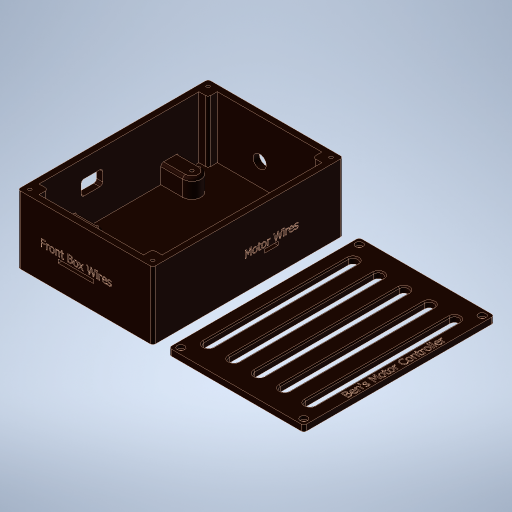
# Autodesk Inventor part: Back Circuit Box
Saved by Autodesk Inventor 2024 (Build 280153000, 153)
## iProperties
Created: 2024-02-09
Part Number: Back Circuit Box
Material: PC/ABS Plastic
Document SubType Name: Modeling
Designer: himmelb
Density: 1.1 g/cm^3
Appearance: Smooth - Dark Brown
Author: himmelb
Autodesk Inventor part; units mm, degrees
(part 1 of 3)
ref_plane "YZ Plane" through (0, 0, 0) normal (1, 0, 0) x (0, 1, 0)
ref_plane "XZ Plane" through (0, 0, 0) normal (0, 1, 0) x (-1, 0, 0)
ref_plane "XY Plane" through (0, 0, 0) normal (0, 0, 1) x (1, 0, 0)
sketch "Sketch1" plane through (0, 0, 0) normal (0, 1, 0) x (-1, 0, 0)
  line L0 (0, 0) -> (110, 0)
  line L1 (110, 0) -> (110, -155)
  line L2 (110, -155) -> (0, -155)
  line L3 (0, -155) -> (0, 0)
  dimension "d0" = 155
  dimension "d1" = 110
  constraints: 8 end point, 2 parallel, 1 horizontal, 1 perpendicular
  measures "d0" distance of L0.end L1.end
  measures "d1" distance of L1.end L2.end
extrude "Extrusion1" add sketch "Sketch1" along normal blind 55
shell "Shell1" thickness 5 removed faces 1 at (-36.6667, 55, -51.6667)
sketch "Sketch2" plane through (0, 0, 0) normal (0, -1, 0) x (1, 0, 0)
  line L0 (12.8693, 0) -> (122.8693, 0)
  line L1 (122.8693, 0) -> (122.8693, -155)
  line L2 (122.8693, -155) -> (12.8693, -155)
  line L3 (12.8693, -155) -> (12.8693, 0)
  point P0 (0, 0)
  dimension "d5" = 110
  dimension "d6" = 155
  constraints: 8 end point, 2 parallel, 1 horizontal, 1 perpendicular
  measures "d5" distance of L1.end L2.end
  measures "d6" distance of L0.end L1.end
extrude "Extrusion2" add sketch "Sketch2" against normal blind 5
sketch "Sketch3" plane through (0, 5, 0) normal (0, 1, 0) x (1, 0, 0)
  line L0 (12.8693, 155) -> (12.8693, 0) projected
  line L1 (105.3693, 18.75) -> (105.3693, 136.25)
  line L2 (112.8693, 136.25) -> (112.8693, 18.75)
  arc A0 (112.8693, 136.25) -> (105.3693, 136.25) centre (109.1193, 136.25) ccw
  arc A1 (105.3693, 18.75) -> (112.8693, 18.75) centre (109.1193, 18.75) ccw
  line L3 (22.8693, 136.25) -> (22.8693, 18.75)
  line L4 (122.8693, 0) -> (122.8693, 155) projected
  circle A2 centre (17.8693, 5) radius 1.335
  circle A3 centre (117.8693, 5) radius 1.335
  circle A4 centre (17.8693, 150) radius 1.335
  circle A5 centre (117.8693, 150) radius 1.335
  line L5 (92.2443, 18.75) -> (92.2443, 136.25)
  arc A6 (92.2443, 136.25) -> (84.7443, 136.25) centre (88.4943, 136.25) ccw
  line L6 (84.7443, 136.25) -> (84.7443, 18.75)
  arc A7 (84.7443, 18.75) -> (92.2443, 18.75) centre (88.4943, 18.75) ccw
  line L7 (71.6193, 18.75) -> (71.6193, 136.25)
  line L8 (122.8693, 155) -> (12.8693, 155) projected
  arc A8 (71.6193, 136.25) -> (67.8693, 140) centre (67.8693, 136.25) ccw
  arc A9 (67.8693, 15) -> (71.6193, 18.75) centre (67.8693, 18.75) ccw
  line L9 (12.8693, 0) -> (122.8693, 0) projected
  line L10 (30.3693, 18.75) -> (30.3693, 136.25)
  line L11 (22.8693, 136.25) -> (22.8693, 18.75)
  arc A10 (30.3693, 136.25) -> (22.8693, 136.25) centre (26.6193, 136.25) ccw
  arc A11 (22.8693, 18.75) -> (30.3693, 18.75) centre (26.6193, 18.75) ccw
  line L12 (43.4943, 18.75) -> (43.4943, 136.25)
  arc A12 (50.9943, 136.25) -> (43.4943, 136.25) centre (47.2443, 136.25) ccw
  line L13 (50.9943, 136.25) -> (50.9943, 18.75)
  arc A13 (43.4943, 18.75) -> (50.9943, 18.75) centre (47.2443, 18.75) ccw
  line L14 (64.1193, 18.75) -> (64.1193, 136.25)
  arc A14 (67.8693, 140) -> (64.1193, 136.25) centre (67.8693, 136.25) ccw
  arc A15 (64.1193, 18.75) -> (67.8693, 15) centre (67.8693, 18.75) ccw
  point P0 (0, 0)
  dimension "d39" = 10
  dimension "d40" = 117.5
  dimension "d41" = 10
  dimension "d45" = 2.67
  dimension "d47" = 5
  dimension "d49" = 5
  dimension "d52" = 5
  dimension "d53" = 5
  dimension "d55" = 2.67
  dimension "d167" = 13.125
  dimension "d168" = 7.5
  dimension "d169" = 13.125
  constraints: 24 point on circle, 22 end point, 16 centre point, 3 vertical
  measures "d39" distance between parallel lines of L4 L2
  measures "d40" distance of L3.start L3.end
  measures "d41" distance between parallel lines of L0 L3
  measures "d45" diameter of A2
  measures "d47" distance from line of A2.centre L0
  measures "d49" distance from line of L4 A3.centre
  measures "d52" distance from line of L0 A4.centre
  measures "d53" distance from line of L4 A5.centre
  measures "d55" diameter of A5
  measures "d167" distance of L1.start L5.start
  measures "d168" diameter of A6
  measures "d169" distance of L6.end L7.start
extrude "Extrusion3" cut sketch "Sketch3" against normal through all contours L1 A0 L2 A1 | A10 L10 A11 L3 | A2 | A3 | A4 | A5 | A7 L6 A6 L5 | A9 A15 L14 A14 A8 L7 | L12 A12 L13 A13
sketch "Sketch4" plane through (0, 5, 0) normal (0, 1, 0) x (1, 0, 0)
  line L0 (115.5683, 32.7918) -> (115.5683, 122.2082) construction
  line L1 (115.5683, 122.2082) -> (120.8693, 122.2082) construction
  line L2 (120.8693, 122.2082) -> (120.8693, 32.7918) construction
  line L3 (120.8693, 32.7918) -> (115.5683, 32.7918) construction
  line L4 (122.8693, 0) -> (122.8693, 155) projected
  spline S0 degree 2 poles (119.4465, 41.7917) (119.8938, 41.7917) (120.5794, 41.4514) (120.8031, 41.1694) knots 0 0 0 1 2 2 2
  spline S1 degree 2 poles (120.8031, 41.1694) (121.0656, 40.829) (121.2893, 40.0559) (121.2893, 39.4433) knots 0 0 0 1 2 2 2
  line L5 (121.2893, 39.4433) -> (121.2893, 37.722)
  line L6 (121.2893, 37.722) -> (115.2893, 37.722)
  line L7 (115.2893, 37.722) -> (115.2893, 39.312)
  spline S2 degree 2 poles (115.2893, 39.312) (115.2893, 39.9538) (115.3719, 40.5956) (115.5324, 40.8874) knots 0 0 0 1 2 2 2
  spline S3 degree 2 poles (115.5324, 40.8874) (115.7026, 41.2131) (116.2617, 41.5097) (116.641, 41.5097) knots 0 0 0 1 2 2 2
  spline S4 degree 2 poles (116.641, 41.5097) (117.064, 41.5097) (117.735, 41.0624) (117.9246, 40.6686) knots 0 0 0 1 2 2 2
  line L8 (117.9246, 40.6686) -> (117.9538, 40.6686)
  spline S5 degree 2 poles (117.9538, 40.6686) (118.0997, 41.2034) (118.8728, 41.7917) (119.4465, 41.7917) knots 0 0 0 1 2 2 2
  spline S6 degree 2 poles (119.4805, 40.9603) (119.1402, 40.9603) (118.7026, 40.7658) (118.547, 40.4741) knots 0 0 0 1 2 2 2
  spline S7 degree 2 poles (118.547, 40.4741) (118.4497, 40.2844) (118.3914, 39.8371) (118.3914, 39.4238) knots 0 0 0 1 2 2 2
  line L9 (118.3914, 39.4238) -> (118.3914, 38.5194)
  line L10 (118.3914, 38.5194) -> (120.6086, 38.5194)
  line L11 (120.6086, 38.5194) -> (120.6086, 39.1661)
  spline S8 degree 2 poles (120.6086, 39.1661) (120.6086, 39.6912) (120.5113, 40.2942) (120.3557, 40.5275) knots 0 0 0 1 2 2 2
  spline S9 degree 2 poles (120.3557, 40.5275) (120.1953, 40.7512) (119.7966, 40.9603) (119.4805, 40.9603) knots 0 0 0 1 2 2 2
  spline S10 degree 2 poles (116.7528, 40.6783) (116.5389, 40.6783) (116.218, 40.5324) (116.1256, 40.372) knots 0 0 0 1 2 2 2
  spline S11 degree 2 poles (116.1256, 40.372) (116.0186, 40.1775) (115.97, 39.7058) (115.97, 39.2828) knots 0 0 0 1 2 2 2
  line L12 (115.97, 39.2828) -> (115.97, 38.5194)
  line L13 (115.97, 38.5194) -> (117.7253, 38.5194)
  line L14 (117.7253, 38.5194) -> (117.7253, 39.4238)
  spline S12 degree 2 poles (117.7253, 39.4238) (117.7253, 39.7982) (117.6475, 40.1532) (117.5259, 40.3428) knots 0 0 0 1 2 2 2
  spline S13 degree 2 poles (117.5259, 40.3428) (117.4092, 40.5275) (117.0348, 40.6783) (116.7528, 40.6783) knots 0 0 0 1 2 2 2
  spline S14 degree 2 poles (121.3914, 44.4805) (121.3914, 43.4011) (120.1807, 42.2147) (119.0624, 42.2147) knots 0 0 0 1 2 2 2
  spline S15 degree 2 poles (119.0624, 42.2147) (117.9635, 42.2147) (116.6604, 43.3671) (116.6604, 44.2958) knots 0 0 0 1 2 2 2
  spline S16 degree 2 poles (116.6604, 44.2958) (116.6604, 44.7139) (116.9036, 45.3606) (117.1612, 45.5989) knots 0 0 0 1 2 2 2
  spline S17 degree 2 poles (117.1612, 45.5989) (117.4189, 45.842) (118.1629, 46.0997) (118.7026, 46.0997) knots 0 0 0 1 2 2 2
  line L15 (118.7026, 46.0997) -> (119.1159, 46.0997)
  line L16 (119.1159, 46.0997) -> (119.1159, 42.983)
  spline S18 degree 2 poles (119.1159, 42.983) (119.8987, 42.983) (120.7301, 43.7707) (120.7301, 44.4708) knots 0 0 0 1 2 2 2
  spline S19 degree 2 poles (120.7301, 44.4708) (120.7301, 44.7188) (120.6183, 45.2002) (120.5308, 45.3946) knots 0 0 0 1 2 2 2
  spline S20 degree 2 poles (120.5308, 45.3946) (120.4335, 45.5989) (120.2634, 45.8809) (120.1856, 45.9733) knots 0 0 0 1 2 2 2
  line L17 (120.1856, 45.9733) -> (120.1856, 46.017)
  line L18 (120.1856, 46.017) -> (121.0121, 46.017)
  spline S21 degree 2 poles (121.0121, 46.017) (121.0656, 45.8857) (121.2212, 45.487) (121.265, 45.3314) knots 0 0 0 1 2 2 2
  spline S22 degree 2 poles (121.265, 45.3314) (121.3282, 45.1126) (121.3914, 44.7528) (121.3914, 44.4805) knots 0 0 0 1 2 2 2
  spline S23 degree 2 poles (118.5373, 45.3606) (118.2309, 45.3509) (117.7836, 45.2245) (117.6329, 45.1029) knots 0 0 0 1 2 2 2
  spline S24 degree 2 poles (117.6329, 45.1029) (117.4627, 44.9716) (117.2828, 44.5583) (117.2828, 44.252) knots 0 0 0 1 2 2 2
  spline S25 degree 2 poles (117.2828, 44.252) (117.2828, 43.9506) (117.4627, 43.5275) (117.6377, 43.3525) knots 0 0 0 1 2 2 2
  spline S26 degree 2 poles (117.6377, 43.3525) (117.8177, 43.1823) (118.2504, 43.0073) (118.5373, 42.983) knots 0 0 0 1 2 2 2
  line L19 (118.5373, 42.983) -> (118.5373, 45.3606)
  line L20 (121.2893, 50.4028) -> (121.2893, 49.6442)
  line L21 (121.2893, 49.6442) -> (118.722, 49.6442)
  spline S27 degree 2 poles (118.722, 49.6442) (118.4108, 49.6442) (117.876, 49.5859) (117.7155, 49.4984) knots 0 0 0 1 2 2 2
  spline S28 degree 2 poles (117.7155, 49.4984) (117.5454, 49.406) (117.38, 49.0754) (117.38, 48.7934) knots 0 0 0 1 2 2 2
  spline S29 degree 2 poles (117.38, 48.7934) (117.38, 48.5113) (117.6815, 47.9133) (117.9246, 47.6264) knots 0 0 0 1 2 2 2
  line L22 (117.9246, 47.6264) -> (121.2893, 47.6264)
  line L23 (121.2893, 47.6264) -> (121.2893, 46.8679)
  line L24 (121.2893, 46.8679) -> (116.7869, 46.8679)
  line L25 (116.7869, 46.8679) -> (116.7869, 47.6264)
  line L26 (116.7869, 47.6264) -> (117.2877, 47.6264)
  spline S30 degree 2 poles (117.2877, 47.6264) (116.9813, 47.9668) (116.6604, 48.6232) (116.6604, 48.9927) knots 0 0 0 1 2 2 2
  spline S31 degree 2 poles (116.6604, 48.9927) (116.6604, 49.654) (117.5356, 50.4028) (118.3671, 50.4028) knots 0 0 0 1 2 2 2
  line L27 (118.3671, 50.4028) -> (121.2893, 50.4028)
  line L28 (115.0219, 52.2358) -> (117.3557, 52.0608)
  line L29 (117.3557, 52.0608) -> (117.3557, 51.5162)
  line L30 (117.3557, 51.5162) -> (115.0219, 51.3412)
  line L31 (115.0219, 51.3412) -> (115.0219, 52.2358)
  spline S32 degree 2 poles (121.3963, 54.4238) (121.3963, 53.9716) (121.1531, 53.1888) (121.017, 52.9311) knots 0 0 0 1 2 2 2
  line L32 (121.017, 52.9311) -> (120.1661, 52.9311)
  line L33 (120.1661, 52.9311) -> (120.1661, 52.97)
  spline S33 degree 2 poles (120.1661, 52.97) (120.2439, 53.0673) (120.4287, 53.3298) (120.5308, 53.5486) knots 0 0 0 1 2 2 2
  spline S34 degree 2 poles (120.5308, 53.5486) (120.6232, 53.7382) (120.7593, 54.205) (120.7593, 54.453) knots 0 0 0 1 2 2 2
  spline S35 degree 2 poles (120.7593, 54.453) (120.7593, 54.6329) (120.6766, 55.0462) (120.6086, 55.1434) knots 0 0 0 1 2 2 2
  spline S36 degree 2 poles (120.6086, 55.1434) (120.5162, 55.2844) (120.3071, 55.4109) (120.0932, 55.4109) knots 0 0 0 1 2 2 2
  spline S37 degree 2 poles (120.0932, 55.4109) (119.8258, 55.4109) (119.5486, 55.1191) (119.4562, 54.7447) knots 0 0 0 1 2 2 2
  spline S38 degree 2 poles (119.4562, 54.7447) (119.4222, 54.5989) (119.3249, 54.1321) (119.2715, 53.9327) knots 0 0 0 1 2 2 2
  spline S39 degree 2 poles (119.2715, 53.9327) (119.1207, 53.4173) (118.4984, 52.9506) (118.0559, 52.9506) knots 0 0 0 1 2 2 2
  spline S40 degree 2 poles (118.0559, 52.9506) (117.4433, 52.9506) (116.6799, 53.8695) (116.6799, 54.628) knots 0 0 0 1 2 2 2
  spline S41 degree 2 poles (116.6799, 54.628) (116.6799, 55.0024) (116.8647, 55.7609) (117.0057, 56.0186) knots 0 0 0 1 2 2 2
  line L34 (117.0057, 56.0186) -> (117.8177, 56.0186)
  line L35 (117.8177, 56.0186) -> (117.8177, 55.9797)
  spline S42 degree 2 poles (117.8177, 55.9797) (117.5843, 55.688) (117.3168, 54.9781) (117.3168, 54.6134) knots 0 0 0 1 2 2 2
  spline S43 degree 2 poles (117.3168, 54.6134) (117.3168, 54.2391) (117.6329, 53.7237) (117.9489, 53.7237) knots 0 0 0 1 2 2 2
  spline S44 degree 2 poles (117.9489, 53.7237) (118.2358, 53.7237) (118.513, 54.03) (118.6005, 54.3703) knots 0 0 0 1 2 2 2
  spline S45 degree 2 poles (118.6005, 54.3703) (118.6442, 54.5357) (118.7318, 54.9538) (118.7852, 55.1823) knots 0 0 0 1 2 2 2
  spline S46 degree 2 poles (118.7852, 55.1823) (118.9117, 55.6783) (119.4903, 56.184) (119.9911, 56.184) knots 0 0 0 1 2 2 2
  spline S47 degree 2 poles (119.9911, 56.184) (120.2828, 56.184) (120.7982, 55.9554) (120.9878, 55.7318) knots 0 0 0 1 2 2 2
  spline S48 degree 2 poles (120.9878, 55.7318) (121.1872, 55.4935) (121.3963, 54.8857) (121.3963, 54.4238) knots 0 0 0 1 2 2 2
  line L36 (121.2893, 64.6686) -> (121.2893, 63.8711)
  line L37 (121.2893, 63.8711) -> (116.1207, 63.8711)
  line L38 (116.1207, 63.8711) -> (119.6361, 62.3055)
  line L39 (119.6361, 62.3055) -> (119.6361, 61.8193)
  line L40 (119.6361, 61.8193) -> (116.1207, 60.2682)
  line L41 (116.1207, 60.2682) -> (121.2893, 60.2682)
  line L42 (121.2893, 60.2682) -> (121.2893, 59.5243)
  line L43 (121.2893, 59.5243) -> (115.2893, 59.5243)
  line L44 (115.2893, 59.5243) -> (115.2893, 60.6134)
  line L45 (115.2893, 60.6134) -> (118.6296, 62.111)
  line L46 (118.6296, 62.111) -> (115.2893, 63.56)
  line L47 (115.2893, 63.56) -> (115.2893, 64.6686)
  line L48 (115.2893, 64.6686) -> (121.2893, 64.6686)
  spline S49 degree 2 poles (119.0381, 69.5259) (120.1758, 69.5259) (121.4157, 68.4319) (121.4157, 67.5178) knots 0 0 0 1 2 2 2
  spline S50 degree 2 poles (121.4157, 67.5178) (121.4157, 66.5794) (120.1369, 65.5049) (119.0381, 65.5049) knots 0 0 0 1 2 2 2
  spline S51 degree 2 poles (119.0381, 65.5049) (117.91, 65.5049) (116.6604, 66.6134) (116.6604, 67.5178) knots 0 0 0 1 2 2 2
  spline S52 degree 2 poles (116.6604, 67.5178) (116.6604, 68.4319) (117.9052, 69.5259) (119.0381, 69.5259) knots 0 0 0 1 2 2 2
  spline S53 degree 2 poles (119.0381, 68.7431) (118.1629, 68.7431) (117.312, 68.1062) (117.312, 67.5178) knots 0 0 0 1 2 2 2
  spline S54 degree 2 poles (117.312, 67.5178) (117.312, 66.9295) (118.1629, 66.2877) (119.0381, 66.2877) knots 0 0 0 1 2 2 2
  spline S55 degree 2 poles (119.0381, 66.2877) (119.889, 66.2877) (120.7642, 66.9295) (120.7642, 67.5178) knots 0 0 0 1 2 2 2
  spline S56 degree 2 poles (120.7642, 67.5178) (120.7642, 68.1013) (119.9036, 68.7431) (119.0381, 68.7431) knots 0 0 0 1 2 2 2
  spline S57 degree 2 poles (121.3768, 71.6653) (121.3768, 71.0478) (120.6718, 70.3525) (119.9084, 70.3525) knots 0 0 0 1 2 2 2
  line L49 (119.9084, 70.3525) -> (117.4141, 70.3525)
  line L50 (117.4141, 70.3525) -> (117.4141, 69.842)
  line L51 (117.4141, 69.842) -> (116.7869, 69.842)
  line L52 (116.7869, 69.842) -> (116.7869, 70.3525)
  line L53 (116.7869, 70.3525) -> (115.4935, 70.3525)
  line L54 (115.4935, 70.3525) -> (115.4935, 71.111)
  line L55 (115.4935, 71.111) -> (116.7869, 71.111)
  line L56 (116.7869, 71.111) -> (116.7869, 72.5065)
  line L57 (116.7869, 72.5065) -> (117.4141, 72.5065)
  line L58 (117.4141, 72.5065) -> (117.4141, 71.111)
  line L59 (117.4141, 71.111) -> (119.5583, 71.111)
  spline S58 degree 2 poles (119.5583, 71.111) (119.8987, 71.111) (120.2731, 71.1353) (120.4335, 71.218) knots 0 0 0 1 2 2 2
  spline S59 degree 2 poles (120.4335, 71.218) (120.5745, 71.2861) (120.7155, 71.5924) (120.7155, 71.8549) knots 0 0 0 1 2 2 2
  spline S60 degree 2 poles (120.7155, 71.8549) (120.7155, 72.0397) (120.6037, 72.3849) (120.5697, 72.4627) knots 0 0 0 1 2 2 2
  line L60 (120.5697, 72.4627) -> (120.5697, 72.5065)
  line L61 (120.5697, 72.5065) -> (121.2504, 72.5065)
  spline S61 degree 2 poles (121.2504, 72.5065) (121.3087, 72.2925) (121.3768, 71.8549) (121.3768, 71.6653) knots 0 0 0 1 2 2 2
  spline S62 degree 2 poles (119.0381, 76.7658) (120.1758, 76.7658) (121.4157, 75.6718) (121.4157, 74.7577) knots 0 0 0 1 2 2 2
  spline S63 degree 2 poles (121.4157, 74.7577) (121.4157, 73.8193) (120.1369, 72.7447) (119.0381, 72.7447) knots 0 0 0 1 2 2 2
  spline S64 degree 2 poles (119.0381, 72.7447) (117.91, 72.7447) (116.6604, 73.8533) (116.6604, 74.7577) knots 0 0 0 1 2 2 2
  spline S65 degree 2 poles (116.6604, 74.7577) (116.6604, 75.6718) (117.9052, 76.7658) (119.0381, 76.7658) knots 0 0 0 1 2 2 2
  spline S66 degree 2 poles (119.0381, 75.983) (118.1629, 75.983) (117.312, 75.346) (117.312, 74.7577) knots 0 0 0 1 2 2 2
  spline S67 degree 2 poles (117.312, 74.7577) (117.312, 74.1694) (118.1629, 73.5275) (119.0381, 73.5275) knots 0 0 0 1 2 2 2
  spline S68 degree 2 poles (119.0381, 73.5275) (119.889, 73.5275) (120.7642, 74.1694) (120.7642, 74.7577) knots 0 0 0 1 2 2 2
  spline S69 degree 2 poles (120.7642, 74.7577) (120.7642, 75.3412) (119.9036, 75.983) (119.0381, 75.983) knots 0 0 0 1 2 2 2
  line L62 (117.5988, 79.9311) -> (117.5988, 79.8922)
  spline S70 degree 2 poles (117.5988, 79.8922) (117.5745, 79.8047) (117.5648, 79.6151) (117.5648, 79.4838) knots 0 0 0 1 2 2 2
  spline S71 degree 2 poles (117.5648, 79.4838) (117.5648, 79.1775) (117.8322, 78.5746) (118.0948, 78.3023) knots 0 0 0 1 2 2 2
  line L63 (118.0948, 78.3023) -> (121.2893, 78.3023)
  line L64 (121.2893, 78.3023) -> (121.2893, 77.5438)
  line L65 (121.2893, 77.5438) -> (116.7869, 77.5438)
  line L66 (116.7869, 77.5438) -> (116.7869, 78.3023)
  line L67 (116.7869, 78.3023) -> (117.4578, 78.3023)
  spline S72 degree 2 poles (117.4578, 78.3023) (117.0883, 78.7156) (116.7869, 79.3331) (116.7869, 79.6248) knots 0 0 0 1 2 2 2
  spline S73 degree 2 poles (116.7869, 79.6248) (116.7869, 79.7415) (116.7966, 79.8582) (116.8112, 79.9311) knots 0 0 0 1 2 2 2
  line L68 (116.8112, 79.9311) -> (117.5988, 79.9311)
  spline S74 degree 2 poles (121.3963, 85.4984) (121.3963, 84.9149) (121.0024, 83.9279) (120.6086, 83.5681) knots 0 0 0 1 2 2 2
  spline S75 degree 2 poles (120.6086, 83.5681) (120.2196, 83.2083) (119.0527, 82.8144) (118.2941, 82.8144) knots 0 0 0 1 2 2 2
  spline S76 degree 2 poles (118.2941, 82.8144) (117.5405, 82.8144) (116.4222, 83.1985) (116.0089, 83.5632) knots 0 0 0 1 2 2 2
  spline S77 degree 2 poles (116.0089, 83.5632) (115.6053, 83.923) (115.1823, 84.9052) (115.1823, 85.513) knots 0 0 0 1 2 2 2
  spline S78 degree 2 poles (115.1823, 85.513) (115.1823, 85.8144) (115.2698, 86.3444) (115.3379, 86.5681) knots 0 0 0 1 2 2 2
  spline S79 degree 2 poles (115.3379, 86.5681) (115.4011, 86.7626) (115.581, 87.1661) (115.688, 87.3655) knots 0 0 0 1 2 2 2
  line L69 (115.688, 87.3655) -> (116.6507, 87.3655)
  line L70 (116.6507, 87.3655) -> (116.6507, 87.3023)
  spline S80 degree 2 poles (116.6507, 87.3023) (116.5535, 87.1953) (116.2812, 86.8647) (116.1499, 86.6264) knots 0 0 0 1 2 2 2
  spline S81 degree 2 poles (116.1499, 86.6264) (116.0235, 86.3979) (115.863, 85.8582) (115.863, 85.5081) knots 0 0 0 1 2 2 2
  spline S82 degree 2 poles (115.863, 85.5081) (115.863, 85.124) (116.1791, 84.4384) (116.4805, 84.1807) knots 0 0 0 1 2 2 2
  spline S83 degree 2 poles (116.4805, 84.1807) (116.7869, 83.9279) (117.7155, 83.6459) (118.2941, 83.6459) knots 0 0 0 1 2 2 2
  spline S84 degree 2 poles (118.2941, 83.6459) (118.9117, 83.6459) (119.8014, 83.9425) (120.1078, 84.2002) knots 0 0 0 1 2 2 2
  spline S85 degree 2 poles (120.1078, 84.2002) (120.4044, 84.453) (120.7058, 85.1288) (120.7058, 85.5081) knots 0 0 0 1 2 2 2
  spline S86 degree 2 poles (120.7058, 85.5081) (120.7058, 85.8533) (120.5356, 86.4417) (120.4092, 86.6702) knots 0 0 0 1 2 2 2
  spline S87 degree 2 poles (120.4092, 86.6702) (120.2828, 86.889) (120.0202, 87.2147) (119.9279, 87.3071) knots 0 0 0 1 2 2 2
  line L71 (119.9279, 87.3071) -> (119.9279, 87.3655)
  line L72 (119.9279, 87.3655) -> (120.8809, 87.3655)
  spline S88 degree 2 poles (120.8809, 87.3655) (120.9732, 87.1661) (121.1434, 86.816) (121.2212, 86.5681) knots 0 0 0 1 2 2 2
  spline S89 degree 2 poles (121.2212, 86.5681) (121.3087, 86.3055) (121.3963, 85.8582) (121.3963, 85.4984) knots 0 0 0 1 2 2 2
  spline S90 degree 2 poles (119.0381, 91.7512) (120.1758, 91.7512) (121.4157, 90.6572) (121.4157, 89.7431) knots 0 0 0 1 2 2 2
  spline S91 degree 2 poles (121.4157, 89.7431) (121.4157, 88.8047) (120.1369, 87.7301) (119.0381, 87.7301) knots 0 0 0 1 2 2 2
  spline S92 degree 2 poles (119.0381, 87.7301) (117.91, 87.7301) (116.6604, 88.8387) (116.6604, 89.7431) knots 0 0 0 1 2 2 2
  spline S93 degree 2 poles (116.6604, 89.7431) (116.6604, 90.6572) (117.9052, 91.7512) (119.0381, 91.7512) knots 0 0 0 1 2 2 2
  spline S94 degree 2 poles (119.0381, 90.9684) (118.1629, 90.9684) (117.312, 90.3314) (117.312, 89.7431) knots 0 0 0 1 2 2 2
  spline S95 degree 2 poles (117.312, 89.7431) (117.312, 89.1548) (118.1629, 88.513) (119.0381, 88.513) knots 0 0 0 1 2 2 2
  spline S96 degree 2 poles (119.0381, 88.513) (119.889, 88.513) (120.7642, 89.1548) (120.7642, 89.7431) knots 0 0 0 1 2 2 2
  spline S97 degree 2 poles (120.7642, 89.7431) (120.7642, 90.3266) (119.9036, 90.9684) (119.0381, 90.9684) knots 0 0 0 1 2 2 2
  line L73 (121.2893, 96.064) -> (121.2893, 95.3055)
  line L74 (121.2893, 95.3055) -> (118.722, 95.3055)
  spline S98 degree 2 poles (118.722, 95.3055) (118.4108, 95.3055) (117.876, 95.2472) (117.7155, 95.1596) knots 0 0 0 1 2 2 2
  spline S99 degree 2 poles (117.7155, 95.1596) (117.5454, 95.0673) (117.38, 94.7366) (117.38, 94.4546) knots 0 0 0 1 2 2 2
  spline S100 degree 2 poles (117.38, 94.4546) (117.38, 94.1726) (117.6815, 93.5746) (117.9246, 93.2877) knots 0 0 0 1 2 2 2
  line L75 (117.9246, 93.2877) -> (121.2893, 93.2877)
  line L76 (121.2893, 93.2877) -> (121.2893, 92.5292)
  line L77 (121.2893, 92.5292) -> (116.7869, 92.5292)
  line L78 (116.7869, 92.5292) -> (116.7869, 93.2877)
  line L79 (116.7869, 93.2877) -> (117.2877, 93.2877)
  spline S101 degree 2 poles (117.2877, 93.2877) (116.9813, 93.628) (116.6604, 94.2844) (116.6604, 94.654) knots 0 0 0 1 2 2 2
  spline S102 degree 2 poles (116.6604, 94.654) (116.6604, 95.3152) (117.5356, 96.064) (118.3671, 96.064) knots 0 0 0 1 2 2 2
  line L80 (118.3671, 96.064) -> (121.2893, 96.064)
  spline S103 degree 2 poles (121.3768, 98.4903) (121.3768, 97.8728) (120.6718, 97.1775) (119.9084, 97.1775) knots 0 0 0 1 2 2 2
  line L81 (119.9084, 97.1775) -> (117.4141, 97.1775)
  line L82 (117.4141, 97.1775) -> (117.4141, 96.6669)
  line L83 (117.4141, 96.6669) -> (116.7869, 96.6669)
  line L84 (116.7869, 96.6669) -> (116.7869, 97.1775)
  line L85 (116.7869, 97.1775) -> (115.4935, 97.1775)
  line L86 (115.4935, 97.1775) -> (115.4935, 97.936)
  line L87 (115.4935, 97.936) -> (116.7869, 97.936)
  line L88 (116.7869, 97.936) -> (116.7869, 99.3314)
  line L89 (116.7869, 99.3314) -> (117.4141, 99.3314)
  line L90 (117.4141, 99.3314) -> (117.4141, 97.936)
  line L91 (117.4141, 97.936) -> (119.5583, 97.936)
  spline S104 degree 2 poles (119.5583, 97.936) (119.8987, 97.936) (120.2731, 97.9603) (120.4335, 98.0429) knots 0 0 0 1 2 2 2
  spline S105 degree 2 poles (120.4335, 98.0429) (120.5745, 98.111) (120.7155, 98.4173) (120.7155, 98.6799) knots 0 0 0 1 2 2 2
  spline S106 degree 2 poles (120.7155, 98.6799) (120.7155, 98.8647) (120.6037, 99.2099) (120.5697, 99.2877) knots 0 0 0 1 2 2 2
  line L92 (120.5697, 99.2877) -> (120.5697, 99.3314)
  line L93 (120.5697, 99.3314) -> (121.2504, 99.3314)
  spline S107 degree 2 poles (121.2504, 99.3314) (121.3087, 99.1175) (121.3768, 98.6799) (121.3768, 98.4903) knots 0 0 0 1 2 2 2
  line L94 (117.5988, 102.278) -> (117.5988, 102.2391)
  spline S108 degree 2 poles (117.5988, 102.2391) (117.5745, 102.1515) (117.5648, 101.9619) (117.5648, 101.8306) knots 0 0 0 1 2 2 2
  spline S109 degree 2 poles (117.5648, 101.8306) (117.5648, 101.5243) (117.8322, 100.9214) (118.0948, 100.6491) knots 0 0 0 1 2 2 2
  line L95 (118.0948, 100.6491) -> (121.2893, 100.6491)
  line L96 (121.2893, 100.6491) -> (121.2893, 99.8906)
  line L97 (121.2893, 99.8906) -> (116.7869, 99.8906)
  line L98 (116.7869, 99.8906) -> (116.7869, 100.6491)
  line L99 (116.7869, 100.6491) -> (117.4578, 100.6491)
  spline S110 degree 2 poles (117.4578, 100.6491) (117.0883, 101.0624) (116.7869, 101.6799) (116.7869, 101.9716) knots 0 0 0 1 2 2 2
  spline S111 degree 2 poles (116.7869, 101.9716) (116.7869, 102.0883) (116.7966, 102.205) (116.8112, 102.278) knots 0 0 0 1 2 2 2
  line L100 (116.8112, 102.278) -> (117.5988, 102.278)
  spline S112 degree 2 poles (119.0381, 106.5664) (120.1758, 106.5664) (121.4157, 105.4724) (121.4157, 104.5583) knots 0 0 0 1 2 2 2
  spline S113 degree 2 poles (121.4157, 104.5583) (121.4157, 103.6199) (120.1369, 102.5454) (119.0381, 102.5454) knots 0 0 0 1 2 2 2
  spline S114 degree 2 poles (119.0381, 102.5454) (117.91, 102.5454) (116.6604, 103.654) (116.6604, 104.5583) knots 0 0 0 1 2 2 2
  spline S115 degree 2 poles (116.6604, 104.5583) (116.6604, 105.4724) (117.9052, 106.5664) (119.0381, 106.5664) knots 0 0 0 1 2 2 2
  spline S116 degree 2 poles (119.0381, 105.7836) (118.1629, 105.7836) (117.312, 105.1467) (117.312, 104.5583) knots 0 0 0 1 2 2 2
  spline S117 degree 2 poles (117.312, 104.5583) (117.312, 103.97) (118.1629, 103.3282) (119.0381, 103.3282) knots 0 0 0 1 2 2 2
  spline S118 degree 2 poles (119.0381, 103.3282) (119.889, 103.3282) (120.7642, 103.97) (120.7642, 104.5583) knots 0 0 0 1 2 2 2
  spline S119 degree 2 poles (120.7642, 104.5583) (120.7642, 105.1418) (119.9036, 105.7836) (119.0381, 105.7836) knots 0 0 0 1 2 2 2
  line L101 (121.2893, 108.1175) -> (121.2893, 107.359)
  line L102 (121.2893, 107.359) -> (115.0219, 107.359)
  line L103 (115.0219, 107.359) -> (115.0219, 108.1175)
  line L104 (115.0219, 108.1175) -> (121.2893, 108.1175)
  line L105 (121.2893, 110.0041) -> (121.2893, 109.2455)
  line L106 (121.2893, 109.2455) -> (115.0219, 109.2455)
  line L107 (115.0219, 109.2455) -> (115.0219, 110.0041)
  line L108 (115.0219, 110.0041) -> (121.2893, 110.0041)
  spline S120 degree 2 poles (121.3914, 113.0721) (121.3914, 111.9927) (120.1807, 110.8063) (119.0624, 110.8063) knots 0 0 0 1 2 2 2
  spline S121 degree 2 poles (119.0624, 110.8063) (117.9635, 110.8063) (116.6604, 111.9587) (116.6604, 112.8874) knots 0 0 0 1 2 2 2
  spline S122 degree 2 poles (116.6604, 112.8874) (116.6604, 113.3055) (116.9036, 113.9522) (117.1612, 114.1904) knots 0 0 0 1 2 2 2
  spline S123 degree 2 poles (117.1612, 114.1904) (117.4189, 114.4335) (118.1629, 114.6912) (118.7026, 114.6912) knots 0 0 0 1 2 2 2
  line L109 (118.7026, 114.6912) -> (119.1159, 114.6912)
  line L110 (119.1159, 114.6912) -> (119.1159, 111.5746)
  spline S124 degree 2 poles (119.1159, 111.5746) (119.8987, 111.5746) (120.7301, 112.3622) (120.7301, 113.0624) knots 0 0 0 1 2 2 2
  spline S125 degree 2 poles (120.7301, 113.0624) (120.7301, 113.3104) (120.6183, 113.7917) (120.5308, 113.9862) knots 0 0 0 1 2 2 2
  spline S126 degree 2 poles (120.5308, 113.9862) (120.4335, 114.1904) (120.2634, 114.4724) (120.1856, 114.5648) knots 0 0 0 1 2 2 2
  line L111 (120.1856, 114.5648) -> (120.1856, 114.6086)
  line L112 (120.1856, 114.6086) -> (121.0121, 114.6086)
  spline S127 degree 2 poles (121.0121, 114.6086) (121.0656, 114.4773) (121.2212, 114.0786) (121.265, 113.923) knots 0 0 0 1 2 2 2
  spline S128 degree 2 poles (121.265, 113.923) (121.3282, 113.7042) (121.3914, 113.3444) (121.3914, 113.0721) knots 0 0 0 1 2 2 2
  spline S129 degree 2 poles (118.5373, 113.9522) (118.2309, 113.9425) (117.7836, 113.816) (117.6329, 113.6945) knots 0 0 0 1 2 2 2
  spline S130 degree 2 poles (117.6329, 113.6945) (117.4627, 113.5632) (117.2828, 113.1499) (117.2828, 112.8436) knots 0 0 0 1 2 2 2
  spline S131 degree 2 poles (117.2828, 112.8436) (117.2828, 112.5421) (117.4627, 112.1191) (117.6377, 111.9441) knots 0 0 0 1 2 2 2
  spline S132 degree 2 poles (117.6377, 111.9441) (117.8177, 111.7739) (118.2504, 111.5989) (118.5373, 111.5746) knots 0 0 0 1 2 2 2
  line L113 (118.5373, 111.5746) -> (118.5373, 113.9522)
  line L114 (117.5988, 117.8468) -> (117.5988, 117.8079)
  spline S133 degree 2 poles (117.5988, 117.8079) (117.5745, 117.7204) (117.5648, 117.5308) (117.5648, 117.3995) knots 0 0 0 1 2 2 2
  spline S134 degree 2 poles (117.5648, 117.3995) (117.5648, 117.0932) (117.8322, 116.4903) (118.0948, 116.218) knots 0 0 0 1 2 2 2
  line L115 (118.0948, 116.218) -> (121.2893, 116.218)
  line L116 (121.2893, 116.218) -> (121.2893, 115.4595)
  line L117 (121.2893, 115.4595) -> (116.7869, 115.4595)
  line L118 (116.7869, 115.4595) -> (116.7869, 116.218)
  line L119 (116.7869, 116.218) -> (117.4578, 116.218)
  spline S135 degree 2 poles (117.4578, 116.218) (117.0883, 116.6313) (116.7869, 117.2488) (116.7869, 117.5405) knots 0 0 0 1 2 2 2
  spline S136 degree 2 poles (116.7869, 117.5405) (116.7869, 117.6572) (116.7966, 117.7739) (116.8112, 117.8468) knots 0 0 0 1 2 2 2
  line L120 (116.8112, 117.8468) -> (117.5988, 117.8468)
  point P0 (0, 0)
  point P1 (120.8693, 77.5)
  point P2 (122.8693, 77.5)
  point P3 (120.8693, 77.5)
  point P4 (122.8693, 77.5)
  dimension "d59" = 2
  dimension "d61" = 0
  constraints: 3 midpoint, 1 coincident, 2 other
  measures "d59" distance between parallel lines of L4 L2
  measures "d61" vertical distance of point (122.869, 77.5) point (120.869, 77.5)
extrude "Extrusion4" cut sketch "Sketch4" against normal blind 1.5
sketch "Sketch5" plane through (0, 5, 0) normal (0, 1, 0) x (1, 0, 0)
  circle A0 centre (17.8693, 5) radius 1.335 projected
  circle A1 centre (17.8693, 5) radius 3
  circle A2 centre (17.8693, 150) radius 1.335 projected
  circle A3 centre (17.8693, 150) radius 3
  circle A4 centre (117.8693, 150) radius 1.335 projected
  circle A5 centre (117.8693, 150) radius 3
  circle A6 centre (117.8693, 5) radius 1.335 projected
  circle A7 centre (117.8693, 5) radius 3
  point P0 (0, 0)
  dimension "d66" = 6
  dimension "d67" = 6
  dimension "d68" = 6
  dimension "d69" = 6
  constraints: 4 centre point, 4 coincident
  measures "d66" diameter of A1
  measures "d67" diameter of A7
  measures "d68" diameter of A5
  measures "d69" diameter of A3
extrude "Extrusion5" cut sketch "Sketch5" against normal blind 2.7 contours A0 | A1 | A2 | A3 | A4 | A5 | A6 | A7
sketch "Sketch6" plane through (-105, 5, -150) normal (0, 1, 0) x (1, 0, 0)
  line L0 (0, 0) -> (100, 0) projected
  line L1 (0, 0) -> (7.5, 0)
  line L2 (7.5, 0) -> (7.5, -7.5)
  line L3 (7.5, -7.5) -> (0, -7.5)
  line L4 (0, -7.5) -> (0, 0)
  line L5 (0, -145) -> (0, 0) projected
  line L6 (100, 0) -> (0, 0)
  line L7 (100, 0) -> (92.5, 0)
  line L8 (92.5, 0) -> (92.5, -7.5)
  line L9 (92.5, -7.5) -> (100, -7.5)
  line L10 (100, -145) -> (100, 0)
  line L11 (100, 0) -> (100, -7.5)
  line L12 (0, -145) -> (7.5, -145)
  line L13 (7.5, -145) -> (7.5, -137.5)
  line L14 (7.5, -137.5) -> (0, -137.5)
  line L15 (0, -137.5) -> (0, -145)
  line L16 (92.5, -137.5) -> (100, -137.5)
  line L17 (92.5, -145) -> (92.5, -137.5)
  line L18 (100, -145) -> (92.5, -145)
  line L19 (100, -145) -> (100, -137.5)
  point P0 (105, -150)
  point P1 (0, -137.5)
  point P2 (7.5, 0)
  point P3 (92.5, 0)
  dimension "d72" = 7.5
  dimension "d73" = 7.5
  constraints: 36 end point, 2 parallel, 1 horizontal, 1 perpendicular, 1 vertical
  measures "d72" distance of L1.end L2.end
  measures "d73" distance of L2.end L3.end
extrude "Extrusion6" add sketch "Sketch6" along normal up to surface (50 mm away)
sketch "Sketch7" plane through (0, 55, 0) normal (0, 1, 0) x (1, 0, 0)
  circle A0 centre (-105, 150) radius 1.335
  circle A1 centre (-5, 150) radius 1.335
  circle A2 centre (-5, 5) radius 1.335
  circle A3 centre (-105, 5) radius 1.335
  line L0 (-110, 155) -> (-110, 0) projected
  line L1 (0, 155) -> (-110, 155) projected
  line L2 (0, 0) -> (0, 155) projected
  line L3 (-110, 0) -> (0, 0) projected
  dimension "d76" = 5
  dimension "d77" = 5
  dimension "d78" = 5
  dimension "d79" = 5
  dimension "d80" = 5
  dimension "d81" = 5
  dimension "d82" = 5
  dimension "d83" = 5
  dimension "d84" = 2.67
  dimension "d85" = 2.67
  dimension "d86" = 2.67
  dimension "d87" = 2.67
  constraints: 4 centre point
  measures "d76" distance from line of L0 A0.centre
  measures "d77" distance from line of L1 A0.centre
  measures "d78" distance from line of L1 A1.centre
  measures "d79" distance from line of L2 A1.centre
  measures "d80" distance from line of L2 A2.centre
  measures "d81" distance from line of L3 A2.centre
  measures "d82" distance from line of L3 A3.centre
  measures "d83" distance from line of L0 A3.centre
  measures "d84" diameter of A3
  measures "d85" diameter of A2
  measures "d86" diameter of A1
  measures "d87" diameter of A0
extrude "Extrusion7" cut sketch "Sketch7" against normal blind 19.8 contours A0 | A1 | A2 | A3
sketch "Sketch8" plane through (-97.5, 5, -5) normal (0, 1, 0) x (1, 0, 0)
  arc A0 (10.3, 106.5) -> (10.3, 121.5) centre (10.3, 114) ccw
  arc A1 (74.7, 121.5) -> (74.7, 106.5) centre (74.7, 114) ccw
  arc A2 (10.3, 23.5) -> (10.3, 38.5) centre (10.3, 31) ccw
  arc A3 (74.7, 38.5) -> (74.7, 23.5) centre (74.7, 31) ccw
  line L0 (97.5, -5) -> (97.5, 150) projected
  line L1 (-12.5, -5) -> (97.5, -5) projected
  line L2 (10.3, 121.5) -> (-7.5, 121.5)
  line L3 (-7.5, 7.5) -> (-7.5, 137.5) projected
  line L4 (10.3, 106.5) -> (-7.5, 106.5)
  line L5 (74.7, 106.5) -> (92.5, 106.5)
  line L6 (92.5, 137.5) -> (92.5, 7.5) projected
  line L7 (74.7, 121.5) -> (92.5, 121.5)
  line L8 (74.7, 38.5) -> (92.5, 38.5)
  line L9 (74.7, 23.5) -> (92.5, 23.5)
  line L10 (10.3, 38.5) -> (-7.5, 38.5)
  line L11 (10.3, 23.5) -> (-7.5, 23.5)
  dimension "d90" = 83
  dimension "d91" = 64.4
  dimension "d92" = 15
  dimension "d93" = 15
  dimension "d94" = 15
  dimension "d95" = 15
  dimension "d96" = 64.4
  dimension "d97" = 83
  dimension "d98" = 22.8
  dimension "d99" = 36
  dimension "d100" = 36
  constraints: 16 end point, 12 point on line, 8 point on circle, 4 centre point, 2 horizontal, 2 parallel, 2 perpendicular, 1 tangent
  measures "d90" distance of A3.centre A1.centre
  measures "d91" distance of A1.centre A0.centre
  measures "d92" diameter of A1
  measures "d93" diameter of A3
  measures "d94" diameter of A0
  measures "d95" diameter of A2
  measures "d96" distance of A3.centre A2.centre
  measures "d97" distance of A0.centre A2.centre
  measures "d98" distance from line of L0 A3.centre
  measures "d99" distance from line of L1 A2.centre
  measures "d100" distance from line of L1 A3.centre
extrude "Extrusion8" add sketch "Sketch8" along normal blind 15
sketch "Sketch9" plane through (-97.5, 20, -5) normal (0, 1, 0) x (1, 0, 0)
  circle A0 centre (10.3, 114) radius 1.335
  line L0 (97.5, 150) -> (-12.5, 150) projected
  line L1 (-12.5, 150) -> (-12.5, -5) projected
  circle A1 centre (74.7, 114) radius 1.335
  circle A2 centre (10.3, 31) radius 1.335
  circle A3 centre (74.7, 31) radius 1.335
  point P0 (97.5, -5)
  point P1 (10.3, 121.5)
  point P2 (10.3, 106.5)
  dimension "d103" = 2.67
  constraints: 4 centre point, 3 coincident
  measures "d103" diameter of A0
extrude "Extrusion9" cut sketch "Sketch9" against normal blind 12
sketch "Sketch10" plane through (0, 0, -155) normal (0, 0, -1) x (-1, 0, 0)
  circle A0 centre (63, 23) radius 5.375
  line L0 (110, 0) -> (110, 55) projected
  line L1 (0, 0) -> (110, 0) projected
  dimension "d106" = 10.75
  dimension "d107" = 47
  dimension "d108" = 23
  constraints: 1 centre point
  measures "d106" diameter of A0
  measures "d107" distance from line of L0 A0.centre
  measures "d108" distance from line of L1 A0.centre
extrude "Extrusion10" cut sketch "Sketch10" against normal up to surface (5 mm away)
sketch "Sketch11" plane through (-110, 0, -155) normal (-1, 0, 0) x (0, 0, 1)
  line L0 (90.75, 40.3) -> (108.25, 40.3)
  line L1 (108.25, 40.3) -> (108.25, 28.3)
  line L2 (108.25, 28.3) -> (90.75, 28.3)
  line L3 (90.75, 28.3) -> (90.75, 40.3)
  line L4 (155, 0) -> (155, 55) projected
  line L5 (0, 0) -> (155, 0) projected
  point P0 (99.5, 40.3)
  point P1 (90.75, 34.3)
  dimension "d111" = 17.5
  dimension "d112" = 12
  dimension "d116" = 55.5
  dimension "d118" = 34.3
  constraints: 8 end point, 2 midpoint, 2 parallel, 1 horizontal, 1 perpendicular
  measures "d111" distance of L0.start L0.end
  measures "d112" distance of L0.end L1.end
  measures "d116" distance from line of L4 point (99.5, 40.3)
  measures "d118" distance from line of L5 point (90.75, 34.3)
extrude "Extrusion11" cut sketch "Sketch11" against normal up to surface (5 mm away)
sketch "Sketch12" plane through (-110, 0, 0) normal (0, 0, 1) x (1, 0, 0)
  line L0 (33.1, 22.45) -> (61.9, 22.45)
  line L1 (61.9, 22.45) -> (61.9, 19.55)
  line L2 (61.9, 19.55) -> (33.1, 19.55)
  line L3 (33.1, 19.55) -> (33.1, 22.45)
  line L4 (0, 0) -> (0, 55) projected
  line L5 (0, 0) -> (110, 0) projected
  point P0 (47.5, 19.55)
  point P1 (33.1, 21)
  dimension "d121" = 28.8
  dimension "d122" = 2.9
  dimension "d123" = 47.5
  dimension "d124" = 21
  constraints: 8 end point, 2 midpoint, 2 parallel, 1 horizontal, 1 perpendicular
  measures "d121" distance of L0.start L0.end
  measures "d122" distance of L0.end L1.end
  measures "d123" distance from line of L4 point (47.5, 19.55)
  measures "d124" distance from line of L5 point (33.1, 21)
extrude "Extrusion12" cut sketch "Sketch12" against normal up to surface (5 mm away)
sketch "Sketch13" plane through (0, 0, 0) normal (1, 0, 0) x (0, 0, -1)
  line L0 (91.15, 22.45) -> (101.85, 22.45)
  line L1 (101.85, 22.45) -> (101.85, 19.55)
  line L2 (101.85, 19.55) -> (91.15, 19.55)
  line L3 (91.15, 19.55) -> (91.15, 22.45)
  line L4 (155, 0) -> (155, 55) projected
  line L5 (0, 0) -> (155, 0) projected
  point P0 (96.5, 22.45)
  point P1 (91.15, 21)
  dimension "d127" = 10.7
  dimension "d128" = 2.9
  dimension "d129" = 58.5
  dimension "d130" = 21
  constraints: 8 end point, 2 midpoint, 2 parallel, 1 horizontal, 1 perpendicular
  measures "d127" distance of L0.start L0.end
  measures "d128" distance of L2.end L0.start
  measures "d129" distance from line of L4 point (96.5, 22.45)
  measures "d130" distance from line of L5 point (91.15, 21)
extrude "Extrusion13" cut sketch "Sketch13" against normal up to surface (5 mm away)
fillet "Fillet1" radius 2.25 28 edges at (122.8693, 2.5, 0) (122.8693, 2.5, -155) (12.8693, 2.5, 0) (-110, 27.5, -155) (0, 27.5, -155) (12.8693, 2.5, -155) (-110, 27.5, 0) (0, 27.5, 0) (-97.5, 30, -142.5) (-12.5, 30, -142.5) (-12.5, 30, -12.5) (-97.5, 30, -12.5) (-96.1, 20, -43.5) (-96.1, 20, -28.5) (-79.7, 20, -36) (-96.1, 20, -126.5) (-96.1, 20, -111.5) (-79.7, 20, -119) (-13.9, 20, -111.5) (-13.9, 20, -126.5) (-30.3, 20, -119) (-13.9, 20, -28.5) (-13.9, 20, -43.5) (-30.3, 20, -36) (-107.5, 28.3, -46.75) (-107.5, 40.3, -46.75) (-107.5, 28.3, -64.25) (-107.5, 40.3, -64.25)
fillet "Fillet3" radius 1 17 edges at (109.1193, 5, -140) (112.8693, 5, -77.5) (109.1193, 5, -15) (105.3693, 5, -77.5) (22.8693, 5, -77.5) (47.2443, 5, -140) (50.9943, 5, -77.5) (47.2443, 5, -15) (43.4943, 5, -77.5) (64.1193, 5, -77.5) (67.8693, 5, -140) (71.6193, 5, -77.5) (67.8693, 5, -15) (84.7443, 5, -77.5) (88.4943, 5, -140) (92.2443, 5, -77.5) (88.4943, 5, -15)